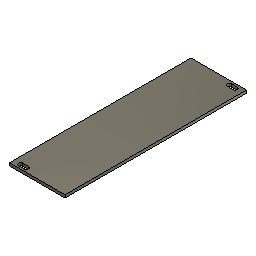
VCF_Abdeckung_v7 (Autodesk Fusion 360 archive; units mm, degrees)
design "Abdeckung_Vorlage_8HP"
Autodesk Fusion 360 part; units mm, degrees
sketch "Skizze1" plane through (0, 0, 0) normal (0, 1, 0) x (1, 0, 0)
  line L0 (0, 0) -> (-39.3, 0)
  line L1 (-39.3, 0) -> (-39.3, -128.5)
  line L2 (-39.3, -128.5) -> (0, -128.5)
  line L3 (0, -128.5) -> (0, 0)
  line L4 (0, 0) -> (-7, 0)
  line L5 (-7, 0) -> (-7, -3)
  line L6 (-39.3, -128.5) -> (-32.3, -128.5)
  line L7 (-32.3, -128.5) -> (-32.3, -125.5)
  line L8 (-7, -3) -> (-9, -3)
  line L9 (-7, -3) -> (-5, -3)
  circle A0 centre (-5, -3) radius 1.5
  circle A1 centre (-9, -3) radius 1.5
  line L10 (-9, -3) -> (-9, -1.5)
  line L11 (-9, -1.5) -> (-5, -1.5)
  line L12 (-9, -4.5) -> (-5, -4.5)
  line L13 (-32.3, -125.5) -> (-34.3, -125.5)
  line L14 (-32.3, -125.5) -> (-30.3, -125.5)
  circle A2 centre (-34.3, -125.5) radius 1.5
  circle A3 centre (-30.3, -125.5) radius 1.5
  line L15 (-34.3, -125.5) -> (-34.3, -124)
  line L16 (-30.3, -125.5) -> (-30.3, -124)
  line L17 (-34.3, -124) -> (-30.3, -124)
  line L18 (-34.3, -125.5) -> (-34.3, -127)
  line L19 (-34.3, -127) -> (-30.3, -127)
  line L20 (0, -128.5) -> (-10, -128.5)
  line L21 (-10, -128.5) -> (-10, -16.5842)
  circle A4 centre (-10, -97.2748) radius 3.5
  line L22 (-10, -97.2748) -> (-10, -76.7748)
  circle A5 centre (-10, -76.7748) radius 3.5
  line L23 (-10, -76.7748) -> (-21.5, -76.7748)
  line L24 (-21.5, -76.7748) -> (-21.5, -39.6569)
  line L25 (-21.5, -76.7748) -> (-21.5, -50.7748)
  line L26 (-21.5, -50.7748) -> (-17.1, -50.7748)
  circle A6 centre (-17.1, -50.7748) radius 3.25
  line L27 (-39.3, 0) -> (-39.3, -25)
  line L28 (-39.3, -25) -> (0, -25)
  line L29 (0, -25) -> (-19.65, -25)
  circle A7 centre (-9.825, -25) radius 3.25
  line L30 (-19.65, -25) -> (-39.3, -25)
  circle A8 centre (-29.475, -25) radius 3.25
  dimension "d1" = 39.3
  dimension "d2" = 128.5
  dimension "d3" = 7
  dimension "d4" = 3
  dimension "d5" = 7
  dimension "d6" = 3
  dimension "d7" = 2
  dimension "d8" = 2
  dimension "d9" = 3
  dimension "d10" = 3
  dimension "d11" = 2
  dimension "d12" = 2
  dimension "d13" = 3
  dimension "d14" = 3
  dimension "d15" = 10
  dimension "d16" = 7
  dimension "d17" = 20.5
  dimension "d18" = 7
  dimension "d19" = 11.5
  dimension "d20" = 26
  dimension "d21" = 4.4
  dimension "d22" = 6.5
  dimension "d23" = 25
  dimension "d24" = 6.5
  dimension "d25" = 6.5
  constraint horizontal L0
  constraint vertical L1
  constraint horizontal L2
  constraint vertical L3
  constraint coincident L0.start L3.end
  constraint perpendicular L3 L4
  constraint perpendicular L0 L5
  constraint perpendicular L1 L6
  constraint perpendicular L2 L7
  constraint perpendicular L5 L8
  constraint perpendicular L5 L9
  constraint coincident L9.end A0.centre
  constraint coincident L8.end A1.centre
  constraint coincident A1 L10.end
  constraint perpendicular L8 L10
  constraint coincident A0 L11.end
  constraint tangent A0 L11
  constraint coincident A1 L12.start
  constraint coincident A0 L12.end
  constraint tangent A0 L12
  constraint parallel L11 L12
  constraint perpendicular L7 L13
  constraint perpendicular L7 L14
  constraint coincident L13.end A2.centre
  constraint coincident L14.end A3.centre
  constraint coincident A2 L15.end
  constraint perpendicular L13 L15
  constraint coincident A3 L16.end
  constraint perpendicular L14 L16
  constraint coincident A2 L18.end
  constraint perpendicular L13 L18
  constraint coincident A3 L19.end
  constraint tangent A3 L19
  constraint perpendicular L3 L20
  constraint perpendicular L12 L21
  constraint coincident L21 A4.centre
  constraint coincident A4.centre L22.start
  constraint parallel L21 L22
  constraint coincident L22.end A5.centre
  constraint perpendicular L22 L23
  constraint perpendicular L23 L24
  constraint perpendicular L23 L25
  constraint perpendicular L3 L26
  constraint coincident L26.end A6.centre
  constraint perpendicular L0 L27
  constraint coincident L3 L28.end
  constraint perpendicular L3 L28
  constraint midpoint L28 L29.end
  constraint midpoint L29 A7.centre
  constraint midpoint L30 A8.centre
  measures "d1" distance of L0.start L0.end
  measures "d2" distance of L0.start L2.end
  measures "d3" distance of L0.start L4.end
  measures "d4" distance of L4.end L5.end
  measures "d5" distance of L1.end L6.end
  measures "d6" distance of L6.end L7.end
  measures "d7" distance of L5.end L8.end
  measures "d8" distance of L5.end L9.end
  measures "d9" diameter of A0
  measures "d10" diameter of A1
  measures "d11" distance of L7.end L13.end
  measures "d12" distance of L7.end L14.end
  measures "d13" diameter of A2
  measures "d14" diameter of A3
  measures "d15" distance of L2.end L20.end
  measures "d16" diameter of A4
  measures "d17" distance of A4.centre L22.end
  measures "d18" diameter of A5
  measures "d19" distance of L22.end L23.end
  measures "d20" distance of L23.end L25.end
  measures "d21" distance of L25.end L26.end
  measures "d22" diameter of A6
  measures "d23" distance of L0.end L27.end
  measures "d24" diameter of A7
  measures "d25" diameter of A8
extrude "Extrusion1" add sketch "Skizze1" along normal blind 2 contours L0 L1 L3 L4 L27 L28 L29 A7 L30 A8 | L2 L3 L20 L21 A4 L22 A5 L28 L29 A7 | L1 L2 L6 L21 A4 L22 A5 L28 L29 A7 L30 A8
sketch "Skizze2" plane through (0, 2, 0) normal (0, 1, 0) x (-1, 0, 0)
  circle A0 centre (9.825, 25) radius 3.25
  arc A1 (9, 1.5) -> (9, 4.5) centre (9, 3) ccw
  line L0 (9, 1.5) -> (5, 1.5)
  arc A2 (5, 4.5) -> (5, 1.5) centre (5, 3) ccw
  line L1 (5, 4.5) -> (9, 4.5)
  arc A3 (34.3, 124) -> (34.3, 127) centre (34.3, 125.5) ccw
  line L2 (34.3, 124) -> (30.3, 124)
  arc A4 (30.3, 127) -> (30.3, 124) centre (30.3, 125.5) ccw
  line L3 (30.3, 127) -> (34.3, 127)
  circle A5 centre (10, 76.7748) radius 3.5
  circle A6 centre (10, 97.2748) radius 3.5
  circle A7 centre (17.1, 50.7748) radius 3.25
  circle A8 centre (29.475, 25) radius 3.25
  line L4 (0, 128.5) -> (0, 0)
  line L5 (0, 0) -> (39.3, 0)
  line L6 (39.3, 0) -> (39.3, 128.5)
  line L7 (39.3, 128.5) -> (0, 128.5)
extrude "Extrusion2" add sketch "Skizze2" against normal blind 2 contours A0 | A5 | A6 | A7 | A8
